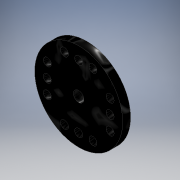
# Autodesk Inventor part: horn
Saved by Autodesk Inventor 2018 (Build 220112000, 112)
## iProperties
Created: 2019-05-28
Part Number: horn
Material: Generic
Document SubType Name: Modeling
Designer: Koki
Density: 1 g/cm^3
Appearance: Black
Author: Koki
Autodesk Inventor part; units mm, degrees
ref_plane "YZ Plane" through (0, 0, 0) normal (1, 0, 0) x (0, 1, 0)
ref_plane "XZ Plane" through (0, 0, 0) normal (0, 1, 0) x (-1, 0, 0)
ref_plane "XY Plane" through (0, 0, 0) normal (0, 0, 1) x (1, 0, 0)
sketch "Sketch1" plane through (0, 0, 0) normal (0, 1, 0) x (-1, 0, 0)
  circle A0 centre (0, 0) radius 10.5
  dimension "d0" = 21
  constraints: 1 centre point, 1 coincident
  measures "d0" diameter of A0
extrude "Extrusion1" add sketch "Sketch1" along normal blind 1.9
sketch "Sketch2" plane through (0, 1.9, 0) normal (0, 1, 0) x (1, 0, 0)
  circle A0 centre (0, 0) radius 4.4
  dimension "d3" = 8.8
  constraints: 1 centre point, 1 coincident
  measures "d3" diameter of A0
extrude "Extrusion2" add sketch "Sketch2" along normal blind 3.5
sketch "Sketch3" plane through (0, 5.4, 0) normal (0, 1, 0) x (1, 0, 0)
  circle A0 centre (0, 0) radius 1.25
  dimension "d6" = 2.5
  constraints: 1 centre point, 1 coincident
  measures "d6" diameter of A0
extrude "Extrusion3" cut sketch "Sketch3" against normal through all
sketch "Sketch4" plane through (0, 0, 0) normal (0, -1, 0) x (1, 0, 0)
  circle A0 centre (7.5, 0) radius 0.95
  circle A1 centre (7.5, -3.4) radius 0.95
  circle A2 centre (7.5, 3.4) radius 0.95
  point P0 (0, 0)
  dimension "d9" = 1.9
  dimension "d10" = 7.5
  dimension "d11" = 1.9
  dimension "d12" = 3.4
  dimension "d13" = 7.5
  dimension "d14" = 1.9
  dimension "d15" = 3.4
  dimension "d16" = 7.5
  constraints: 3 centre point
  measures "d9" diameter of A0
  measures "d10" distance of point (0, 0) A0.centre
  measures "d11" diameter of A1
  measures "d12" distance of A1.centre A0.centre
  measures "d13" horizontal distance of point (0, 0) A1.centre
  measures "d14" diameter of A2
  measures "d15" distance of A0.centre A2.centre
  measures "d16" horizontal distance of point (0, 0) A2.centre
extrude "Extrusion4" cut sketch "Sketch4" against normal through all
pattern_circular "Circular Pattern1" count 4 over 360 about axis through (0, -10, 0) along (0, 1, 0) of "Extrusion4"
equation "\"d13\" = d10"
equation "\"d15\" = d12"
equation "\"d16\" = d10"
body "Solid1"
